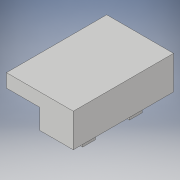
# Autodesk Inventor part: AlignmentPiece
Saved by Autodesk Inventor 2019 (Build 230136000, 136)
## iProperties
Created: 2019-06-19
Part Number: AlignmentPiece
Material: Generic
Document SubType Name: Modeling
Designer: aorfi
Density: 1 g/cm^3
Appearance: Default
Author: aorfi
Autodesk Inventor part; units mm, degrees
ref_plane "YZ Plane" through (0, 0, 0) normal (1, 0, 0) x (0, 1, 0)
ref_plane "XZ Plane" through (0, 0, 0) normal (0, 1, 0) x (-1, 0, 0)
ref_plane "XY Plane" through (0, 0, 0) normal (0, 0, 1) x (1, 0, 0)
sketch "Sketch1" plane through (0, 0, 0) normal (0, 1, 0) x (-1, 0, 0)
  line L0 (-5, 7.5) -> (5, 7.5)
  line L1 (5, 7.5) -> (5, -7.5)
  line L2 (5, -7.5) -> (-5, -7.5)
  line L3 (-5, -7.5) -> (-5, 7.5)
  line L4 (-5, 7.5) -> (5, -7.5) construction
  line L5 (5, 7.5) -> (-5, -7.5) construction
  point P0 (0, 0)
  dimension "d0" = 10
  dimension "d1" = 15
  constraints: 12 end point, 2 midpoint, 2 parallel, 1 horizontal, 1 perpendicular
  measures "d0" distance of L1.end L2.end
  measures "d1" distance of L0.end L1.end
extrude "Extrusion1" add sketch "Sketch1" along normal mid plane 5
sketch "Sketch2" plane through (-5, 2.5, 7.5) normal (0, 0, 1) x (1, 0, 0)
  line L0 (0, 0) -> (0, -5) projected
  line L1 (5, -2) -> (0, -2)
  line L2 (0, -2) -> (0, -5)
  line L3 (0, -5) -> (5, -5)
  line L4 (5, -5) -> (5, -2)
  line L5 (5, -2) -> (0, -5) construction
  line L6 (0, -2) -> (5, -5) construction
  point P0 (5, -2.5)
  point P1 (2.5, -3.5)
  dimension "d4" = 5
  dimension "d13" = 3
  constraints: 12 end point, 2 midpoint, 2 parallel, 1 horizontal, 1 perpendicular
  measures "d4" distance of L1.start L1.end
  measures "d13" distance of L3.end L1.start
extrude "Extrusion2" cut sketch "Sketch2" against normal through all
sketch "Sketch3" plane through (0, -2.5, 0) normal (0, -1, 0) x (1, 0, 0)
  line L0 (3.4, 4.5) -> (1.4, 4.5) construction
  line L1 (1.4, 4.5) -> (1.4, 2.5) construction
  line L2 (1.4, 2.5) -> (3.4, 2.5) construction
  line L3 (3.4, 2.5) -> (3.4, 4.5) construction
  line L4 (3.4, 4.5) -> (1.4, 2.5) construction
  line L5 (1.4, 4.5) -> (3.4, 2.5) construction
  line L6 (3.4, -2.5) -> (1.4, -2.5) construction
  line L7 (1.4, -2.5) -> (1.4, -4.5) construction
  line L8 (1.4, -4.5) -> (3.4, -4.5) construction
  line L9 (3.4, -4.5) -> (3.4, -2.5) construction
  line L10 (3.4, -2.5) -> (1.4, -4.5) construction
  line L11 (1.4, -2.5) -> (3.4, -4.5) construction
  line L12 (2.4, 3.5) -> (2.4, -3.5) construction
  line L13 (3.35, 2.55) -> (1.45, 2.55)
  line L14 (1.45, 2.55) -> (1.45, 4.45)
  line L15 (1.45, 4.45) -> (3.35, 4.45)
  line L16 (3.35, 4.45) -> (3.35, 2.55)
  line L17 (1.45, -2.55) -> (3.35, -2.55)
  line L18 (3.35, -2.55) -> (3.35, -4.45)
  line L19 (3.35, -4.45) -> (1.45, -4.45)
  line L20 (1.45, -4.45) -> (1.45, -2.55)
  line L21 (5, -7.5) -> (5, 7.5) projected
  point P0 (0, 0)
  point P1 (2.4, 0)
  dimension "d7" = 2
  dimension "d8" = 7
  dimension "d11" = 0.05
  dimension "d12" = 0.05
  dimension "d14" = 2.6
  constraints: 42 end point, 8 parallel, 5 midpoint, 4 perpendicular, 3 equal length, 2 horizontal, 1 horizontal alignment, 1 point on line, 1 vertical, 6 other
  measures "d7" distance of L2.end L0.start
  measures "d8" distance of L12.start L12.end
  measures "d11" distance between parallel lines of L2 L13
  measures "d12" distance between parallel lines of L6 L17
  measures "d14" distance between parallel lines of L21 L12
extrude "Extrusion3" add sketch "Sketch3" along normal blind 2
body "Solid1"
